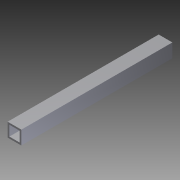
# Autodesk Inventor part: towerbracedraft
Saved by Autodesk Inventor 2011 SP1 (Build 150282100, 282)
## iProperties
Created: 2012-01-18
Part Number: towerbracedraft
Document SubType Name: Modeling
Designer: Christopher
Density: 1 g/cm^3
Author: Christopher
Autodesk Inventor part; units mm, degrees
ref_plane "YZ Plane" through (0, 0, 0) normal (1, 0, 0) x (0, 1, 0)
ref_plane "XZ Plane" through (0, 0, 0) normal (0, 1, 0) x (-1, 0, 0)
ref_plane "XY Plane" through (0, 0, 0) normal (0, 0, 1) x (1, 0, 0)
sketch "Sketch1" plane through (0, 0, 0) normal (0, 0, 1) x (1, 0, 0)
  line L0 (0, 0) -> (25.4, 0)
  line L1 (25.4, 0) -> (25.4, 25.4)
  line L2 (25.4, 25.4) -> (0, 25.4)
  line L3 (0, 25.4) -> (0, 0)
  line L4 (3.175, 3.175) -> (22.225, 3.175)
  line L5 (22.225, 3.175) -> (22.225, 22.225)
  line L6 (22.225, 22.225) -> (3.175, 22.225)
  line L7 (3.175, 22.225) -> (3.175, 3.175)
  dimension "d0" = 25.4
  dimension "d1" = 25.4
  dimension "d2" = 3.175
  constraints: 16 end point, 4 parallel, 2 perpendicular, 1 horizontal, 3 other
  measures "d0" distance of L1.end L2.end
  measures "d1" distance of L0.end L1.end
  measures "d2" distance between parallel lines of L3 L7
extrude "Extrusion1" add sketch "Sketch1" against normal blind 279.4
body "Solid1"
